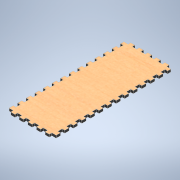
# Autodesk Inventor part: plate_bottom
Saved by Autodesk Inventor 2021 (Build 250183000, 183)
## iProperties
Created: 2021-03-07
Part Number: plate_bottom
Material: Generisch
Document SubType Name: Modeling
Designer: Tilman
Density: 1 g/cm^3
Appearance: Glänzend - Schwarz
Author: Tilman
Autodesk Inventor part; units mm, degrees
ref_plane "YZ Plane" through (0, 0, 0) normal (1, 0, 0) x (0, 1, 0)
ref_plane "XZ Plane" through (0, 0, 0) normal (0, 1, 0) x (-1, 0, 0)
ref_plane "XY Plane" through (0, 0, 0) normal (0, 0, 1) x (1, 0, 0)
sketch "Skizze1" plane through (0, 0, 0) normal (0, 1, 0) x (-1, 0, 0)
  line L0 (0, -3) -> (-5, -3)
  line L1 (-5, -3) -> (-5, 0)
  line L2 (-5, 0) -> (-10, 0)
  line L3 (-10, 0) -> (-10, -3)
  line L4 (-10, -3) -> (-15, -3)
  line L5 (-15, -3) -> (-15, 0)
  line L6 (-15, 0) -> (-20, 0)
  line L7 (-20, 0) -> (-20, -3)
  line L8 (-20, -3) -> (-25, -3)
  line L9 (-25, -3) -> (-25, 0)
  line L10 (-25, 0) -> (-30, 0)
  line L11 (-30, 0) -> (-30, -3)
  line L12 (-30, -3) -> (-35, -3)
  line L13 (-35, -3) -> (-35, 0)
  line L14 (-35, 0) -> (-40, 0)
  line L15 (-40, 0) -> (-40, -3)
  line L16 (-40, -3) -> (-45, -3)
  line L17 (-45, -3) -> (-45, 0)
  line L18 (-45, 0) -> (-50, 0)
  line L19 (-50, 0) -> (-50, -3)
  line L20 (-50, -3) -> (-55, -3)
  line L21 (-55, -3) -> (-55, -8)
  line L22 (-55, -8) -> (-52, -8)
  line L23 (-52, -8) -> (-52, -13)
  line L24 (-52, -13) -> (-55, -13)
  line L25 (-52, -18) -> (-52, -23)
  line L26 (-55, -13) -> (-55, -18)
  line L27 (-55, -18) -> (-52, -18)
  line L28 (-52, -23) -> (-55, -23)
  line L29 (-52, -28) -> (-52, -33)
  line L30 (-55, -23) -> (-55, -28)
  line L31 (-55, -28) -> (-52, -28)
  line L32 (-52, -33) -> (-55, -33)
  line L33 (-52, -38) -> (-52, -43)
  line L34 (-55, -33) -> (-55, -38)
  line L35 (-55, -38) -> (-52, -38)
  line L36 (-52, -43) -> (-55, -43)
  line L37 (-52, -48) -> (-52, -53)
  line L38 (-55, -43) -> (-55, -48)
  line L39 (-55, -48) -> (-52, -48)
  line L40 (-52, -53) -> (-55, -53)
  line L41 (-52, -58) -> (-52, -63)
  line L42 (-55, -53) -> (-55, -58)
  line L43 (-55, -58) -> (-52, -58)
  line L44 (-52, -63) -> (-55, -63)
  line L45 (-52, -68) -> (-52, -73)
  line L46 (-55, -63) -> (-55, -68)
  line L47 (-55, -68) -> (-52, -68)
  line L48 (-52, -73) -> (-55, -73)
  line L49 (-52, -78) -> (-52, -83)
  line L50 (-55, -73) -> (-55, -78)
  line L51 (-55, -78) -> (-52, -78)
  line L52 (-52, -83) -> (-55, -83)
  line L53 (-52, -88) -> (-52, -93)
  line L54 (-55, -83) -> (-55, -88)
  line L55 (-55, -88) -> (-52, -88)
  line L56 (-52, -93) -> (-55, -93)
  line L57 (-52, -98) -> (-52, -103)
  line L58 (-55, -93) -> (-55, -98)
  line L59 (-55, -98) -> (-52, -98)
  line L60 (-52, -103) -> (-55, -103)
  line L61 (-55, -137) -> (-50, -137)
  line L62 (-50, -137) -> (-50, -140)
  line L63 (-50, -140) -> (-45, -140)
  line L64 (-45, -140) -> (-45, -137)
  line L65 (-45, -137) -> (-40, -137)
  line L66 (-40, -140) -> (-35, -140)
  line L67 (-35, -140) -> (-35, -137)
  line L68 (-40, -137) -> (-40, -140)
  line L69 (-35, -137) -> (-30, -137)
  line L70 (-30, -140) -> (-25, -140)
  line L71 (-25, -140) -> (-25, -137)
  line L72 (-30, -137) -> (-30, -140)
  line L73 (-25, -137) -> (-20, -137)
  line L74 (-20, -140) -> (-15, -140)
  line L75 (-15, -140) -> (-15, -137)
  line L76 (-20, -137) -> (-20, -140)
  line L77 (-15, -137) -> (-10, -137)
  line L78 (-10, -140) -> (-5, -140)
  line L79 (-5, -140) -> (-5, -137)
  line L80 (-10, -137) -> (-10, -140)
  line L81 (-5, -137) -> (0, -137)
  line L82 (0, -133) -> (-3, -133)
  line L83 (-3, -133) -> (-3, -128)
  line L84 (-3, -128) -> (0, -128)
  line L85 (0, -128) -> (0, -123)
  line L86 (-52, -108) -> (-52, -113)
  line L87 (-55, -103) -> (-55, -108)
  line L88 (-55, -108) -> (-52, -108)
  line L89 (-52, -113) -> (-55, -113)
  line L90 (-52, -118) -> (-52, -123)
  line L91 (-55, -113) -> (-55, -118)
  line L92 (-55, -118) -> (-52, -118)
  line L93 (-52, -123) -> (-55, -123)
  line L94 (0, -137) -> (0, -133)
  line L95 (-52, -128) -> (-52, -133)
  line L96 (-55, -123) -> (-55, -128)
  line L97 (-55, -128) -> (-52, -128)
  line L98 (-52, -133) -> (-55, -133)
  line L99 (-55, -133) -> (-55, -137)
  line L100 (-3, -123) -> (-3, -118)
  line L101 (0, -118) -> (0, -113)
  line L102 (-3, -118) -> (0, -118)
  line L103 (0, -123) -> (-3, -123)
  line L104 (-3, -113) -> (-3, -108)
  line L105 (0, -108) -> (0, -103)
  line L106 (-3, -108) -> (0, -108)
  line L107 (0, -113) -> (-3, -113)
  line L108 (-3, -103) -> (-3, -98)
  line L109 (0, -98) -> (0, -93)
  line L110 (-3, -98) -> (0, -98)
  line L111 (0, -103) -> (-3, -103)
  line L112 (-3, -93) -> (-3, -88)
  line L113 (0, -88) -> (0, -83)
  line L114 (-3, -88) -> (0, -88)
  line L115 (0, -93) -> (-3, -93)
  line L116 (-3, -83) -> (-3, -78)
  line L117 (0, -78) -> (0, -73)
  line L118 (-3, -78) -> (0, -78)
  line L119 (0, -83) -> (-3, -83)
  line L120 (-3, -73) -> (-3, -68)
  line L121 (0, -68) -> (0, -63)
  line L122 (-3, -68) -> (0, -68)
  line L123 (0, -73) -> (-3, -73)
  line L124 (-3, -63) -> (-3, -58)
  line L125 (0, -58) -> (0, -53)
  line L126 (-3, -58) -> (0, -58)
  line L127 (0, -63) -> (-3, -63)
  line L128 (-3, -53) -> (-3, -48)
  line L129 (0, -48) -> (0, -43)
  line L130 (-3, -48) -> (0, -48)
  line L131 (0, -53) -> (-3, -53)
  line L132 (-3, -43) -> (-3, -38)
  line L133 (0, -38) -> (0, -33)
  line L134 (-3, -38) -> (0, -38)
  line L135 (0, -43) -> (-3, -43)
  line L136 (-3, -33) -> (-3, -28)
  line L137 (0, -28) -> (0, -23)
  line L138 (-3, -28) -> (0, -28)
  line L139 (0, -33) -> (-3, -33)
  line L140 (-3, -23) -> (-3, -18)
  line L141 (0, -18) -> (0, -13)
  line L142 (-3, -18) -> (0, -18)
  line L143 (0, -23) -> (-3, -23)
  line L144 (-3, -13) -> (-3, -8)
  line L145 (0, -8) -> (0, -3)
  line L146 (-3, -8) -> (0, -8)
  line L147 (0, -13) -> (-3, -13)
  point P0 (0, 0)
  dimension "d0" = 3
  dimension "d1" = 5
  dimension "d4" = 10
  dimension "d11" = 10
  dimension "d16" = 140
  dimension "d19" = 10
  dimension "d42" = 10
  constraints: 296 end point, 22 point on line, 18 equal length, 16 perpendicular, 8 horizontal, 4 vertical, 3 collinear, 2 vertical alignment, 1 horizontal alignment, 276 other
  measures "d0" distance of L0.end L1.end
  measures "d1" distance of L0.start L0.end
  measures "d4" distance of L2.end L6.end
  measures "d11" distance of L22.end L25.start
  measures "d16" distance of L18.end L62.end
  measures "d19" distance of L61.start L65.start
  measures "d42" distance of L85.end L101.end
extrude "Extrusion1" add sketch "Skizze1" along normal blind 3
